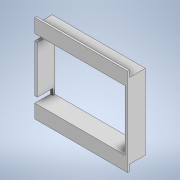
# Autodesk Inventor part: Support_batterie
Saved by Autodesk Inventor 2020.2 (Build 242310000, 310)
## iProperties
Created: 2020-01-14
Part Number: Support_batterie
Material: Générique
Document SubType Name: Modeling
Designer: anton
Density: 1 g/cm^3
Appearance: Par défaut
Author: anton
Autodesk Inventor part; units mm, degrees
ref_plane "YZ Plane" through (0, 0, 0) normal (1, 0, 0) x (0, 1, 0)
ref_plane "XZ Plane" through (0, 0, 0) normal (0, 1, 0) x (-1, 0, 0)
ref_plane "XY Plane" through (0, 0, 0) normal (0, 0, 1) x (1, 0, 0)
sketch "Esquisse1" plane through (0, 0, 0) normal (0, 0, 1) x (1, 0, 0)
  line L0 (-70, 48) -> (70, 48)
  line L1 (70, 48) -> (70, -48)
  line L2 (70, -48) -> (-70, -48)
  line L3 (-70, -48) -> (-70, 48)
  line L4 (74, -60) -> (-74, -60)
  line L5 (-74, -60) -> (-74, 60)
  line L6 (-74, 60) -> (74, 60)
  line L7 (74, 60) -> (74, -60)
  line L8 (74, -60) -> (-74, 60) construction
  line L9 (-74, -60) -> (74, 60) construction
  point P0 (0, 0)
  dimension "d0" = 48
  dimension "d1" = 48
  dimension "d2" = 70
  dimension "d3" = 70
  dimension "d4" = 60
  dimension "d5" = 74
  constraints: 20 end point, 4 parallel, 2 horizontal, 2 midpoint, 2 perpendicular
  measures "d0" distance from line of point (0, 0) L0
  measures "d1" distance from line of point (0, 0) L2
  measures "d2" distance from line of point (0, 0) L3
  measures "d3" distance from line of L1 point (0, 0)
  measures "d4" distance from line of point (0, 0) L6
  measures "d5" distance from line of point (0, 0) L5
extrude "Extrusion1" add sketch "Esquisse1" along normal blind 28
sketch "Esquisse3" plane through (-74, -60, 28) normal (-1, 0, 0) x (0, 0, 1)
  line L0 (-28, 108) -> (0, 108) projected
  line L1 (-28, 48) -> (-28, 4) projected
  line L2 (0, 108) -> (-28, 108)
  line L3 (-28, 108) -> (-28, 98)
  line L4 (-28, 98) -> (0, 98)
  line L5 (0, 98) -> (0, 108)
  line L6 (-28, 12) -> (0, 12) projected
  line L7 (0, 12) -> (-28, 12)
  line L8 (-28, 12) -> (-28, 22)
  line L9 (-28, 22) -> (0, 22)
  line L10 (0, 22) -> (0, 12)
  point P0 (-28, 60)
  point P1 (0, 12)
  point P2 (-28, 22)
  dimension "d10" = 10
  dimension "d11" = 10
  dimension "d12" = 28
  dimension "d13" = 28
  constraints: 16 end point, 4 parallel, 2 horizontal, 2 perpendicular, 2 point on line, 4 other
  measures "d10" distance of L4.end L2.start
  measures "d11" distance of L9.end L7.start
  measures "d12" distance of L8.end L9.end
  measures "d13" distance of L3.end L4.end
extrude "Extrusion3" cut sketch "Esquisse3" against normal blind 10
sketch "Esquisse4" plane through (-74, 60, 28) normal (0, 1, 0) x (1, 0, 0)
  line L0 (148, 28) -> (148, 0) projected
  line L1 (144, 0) -> (4, 0) projected
  line L2 (148, 3) -> (0, 3)
  line L3 (0, 3) -> (0, 0)
  line L4 (0, 0) -> (148, 0)
  line L5 (148, 0) -> (148, 3)
  point P0 (74, 28)
  point P1 (148, 31)
  point P2 (148, 0)
  dimension "d21" = 3
  constraints: 8 end point, 2 parallel, 1 horizontal, 1 perpendicular, 1 point on line
  measures "d21" distance of L2.end L3.end
extrude "Extrusion4" add sketch "Esquisse4" along normal blind 10
sketch "Esquisse5" plane through (-74, -60, 28) normal (0, -1, 0) x (1, 0, 0)
  line L0 (0, 0) -> (144, 0) projected
  line L1 (148, -28) -> (148, -3) projected
  line L2 (0, 0) -> (148, 0)
  line L3 (148, 0) -> (148, -3)
  line L4 (148, -3) -> (0, -3)
  line L5 (0, -3) -> (0, 0)
  point P0 (74, -28)
  point P1 (148, -31)
  point P2 (4, 0)
  point P3 (4, 0)
  dimension "d22" = 3
  constraints: 8 end point, 2 parallel, 1 horizontal, 1 perpendicular, 1 point on line
  measures "d22" distance between parallel lines of L0 L4
extrude "Extrusion5" add sketch "Esquisse5" along normal blind 10
sketch "Esquisse6" plane through (-74, -38, 0) normal (-1, 0, 0) x (0, 0, 1)
  line L0 (0, 86) -> (28, 86) projected
  line L1 (0, -10) -> (28, -10) projected
  line L2 (0, -10) -> (0, -22) projected
  line L3 (0, -10) -> (3, -10)
  line L4 (3, -10) -> (3, 86)
  line L5 (3, 86) -> (0, 86)
  line L6 (0, 86) -> (0, -10)
  point P0 (0, 38)
  dimension "d28" = 3
  constraints: 8 end point, 2 parallel, 1 horizontal, 1 perpendicular, 1 point on line
  measures "d28" distance between parallel lines of L4 L6
extrude "Extrusion6" add sketch "Esquisse6" against normal blind 4
